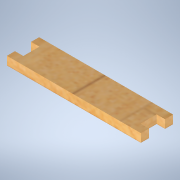
# Autodesk Inventor part: HolzServoHalterHinten
Saved by Autodesk Inventor 2020.3 (Build 243373010, 373A)
## iProperties
Created: 2020-12-10
Part Number: HolzServoHalterHinten
Material: Generisch
Document SubType Name: Modeling
Designer: Stefan
Density: 1 g/cm^3
Appearance: Vorgabe
Author: Stefan
Autodesk Inventor part; units mm, degrees
ref_plane "YZ Plane" through (0, 0, 0) normal (1, 0, 0) x (0, 1, 0)
ref_plane "XZ Plane" through (0, 0, 0) normal (0, 1, 0) x (-1, 0, 0)
ref_plane "XY Plane" through (0, 0, 0) normal (0, 0, 1) x (1, 0, 0)
sketch "Skizze1" plane through (0, 0, 0) normal (0, 1, 0) x (-1, 0, 0)
  line L0 (0, 0) -> (-160, 0)
  line L1 (-160, -38.5) -> (0, -38.5)
  line L2 (0, -9.625) -> (-10, -9.625)
  line L3 (-10, -9.625) -> (-10, -28.875)
  line L4 (-10, -28.875) -> (0, -28.875)
  line L5 (-160, -9.625) -> (-150, -9.625)
  line L6 (-150, -9.625) -> (-150, -28.875)
  line L7 (-150, -28.875) -> (-160, -28.875)
  line L8 (0, -38.5) -> (0, -28.875)
  line L9 (0, -9.625) -> (0, 0)
  line L10 (-160, 0) -> (-160, -9.625)
  line L11 (-160, -28.875) -> (-160, -38.5)
  dimension "d0" = 160
  dimension "d1" = 38.5
  dimension "d2" = 10
  dimension "d3" = 19.25
  dimension "d4" = 10
  dimension "d5" = 19.25
  dimension "d6" = 9.625
  dimension "d7" = 9.625
  constraints: 24 end point, 7 parallel, 4 perpendicular, 3 horizontal, 1 coincident
  measures "d0" distance of L1.end L1.start
  measures "d1" distance of L1.start L0.end
  measures "d2" distance of L4.end L3.end
  measures "d3" distance of L3.end L2.end
  measures "d4" distance of L6.end L7.end
  measures "d5" distance of L5.end L6.end
  measures "d6" distance between parallel lines of L0 L5
  measures "d7" distance between parallel lines of L0 L2
extrude "Extrusion1" add sketch "Skizze1" along normal blind 10
